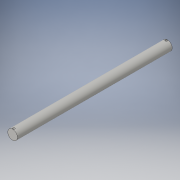
# Autodesk Inventor part: Straw
Saved by Autodesk Inventor 2016 (Build 200138000, 138)
## iProperties
Created: 2017-04-26
Part Number: Straw
Material: Generic
Document SubType Name: Modeling
Designer: wtse3759
Density: 1 g/cm^3
Appearance: Default
Author: wtse3759
Autodesk Inventor part; units mm, degrees
ref_plane "YZ Plane" through (0, 0, 0) normal (1, 0, 0) x (0, 1, 0)
ref_plane "XZ Plane" through (0, 0, 0) normal (0, 1, 0) x (-1, 0, 0)
ref_plane "XY Plane" through (0, 0, 0) normal (0, 0, 1) x (1, 0, 0)
sketch "Sketch1" plane through (0, 0, 0) normal (0, 0, 1) x (1, 0, 0)
  circle A0 centre (0, 0) radius 6.35
  dimension "d0" = 12.7
  constraints: 1 centre point, 1 coincident
  measures "d0" diameter of A0
extrude "Extrusion1" add sketch "Sketch1" along normal blind 203.2
sketch "Sketch4" plane through (0, 0, 0) normal (0, 1, 0) x (-1, 0, 0)
  line L0 (0, 0) -> (0, 1.524)
  line L1 (6.35, 203.2) -> (-6.35, 203.2) projected
  line L2 (0, 203.2) -> (0, 201.676)
  circle A0 centre (0, 201.676) radius 1.27
  circle A1 centre (0, 1.524) radius 1.27
  dimension "d13" = 1.524
  dimension "d15" = 1.524
  dimension "d16" = 2.54
  dimension "d19" = 2.54
  constraints: 4 end point, 2 centre point, 2 coincident, 2 vertical, 1 midpoint
  measures "d13" distance of L0.start L0.end
  measures "d15" distance of L2.start L2.end
  measures "d16" diameter of A0
  measures "d19" diameter of A1
extrude "Extrusion4" cut sketch "Sketch4" along normal mid plane 15.24
body "Solid1"
